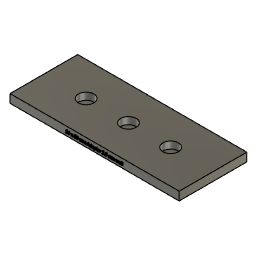
5mm_hydrogel_coverslip_adaptor v2 (Autodesk Fusion 360 design; units mm, degrees)
Autodesk Fusion 360 part; units mm, degrees
sketch "Sketch1" plane through (0, 0, 0) normal (0, 0, 1) x (1, 0, 0)
  line L0 (30, 12) -> (-30, 12)
  line L1 (-30, 12) -> (-30, -12)
  line L2 (-30, -12) -> (30, -12)
  line L3 (30, -12) -> (30, 12)
  line L4 (30, 12) -> (-30, -12) construction
  line L5 (-30, 12) -> (30, -12) construction
  dimension "d1" = 60
  dimension "d2" = 24
  constraint horizontal L0
  constraint perpendicular L0 L1
  constraint parallel L0 L2
  constraint parallel L1 L3
  constraint coincident L4 origin
  constraint coincident L5 origin
  measures "d1" distance of L1.end L2.end
  measures "d2" distance of L0.end L1.end
extrude "Extrude1" add sketch "Sketch1" along normal blind 3
sketch "Sketch2" plane through (0, 0, 3) normal (0, 0, 1) x (-1, 0, 0)
  line L0 (-30, 12) -> (-30, -12)
  line L1 (-30, -12) -> (30, -12)
  line L2 (30, -12) -> (30, 12)
  line L3 (30, 12) -> (-30, 12)
  circle A0 centre (0, 0) radius 2.75
  dimension "d5" = 5.5
  constraint coincident A0.centre origin
  measures "d5" diameter of A0
extrude "Extrude2" cut sketch "Sketch2" against normal blind 2.5 contours A0
sketch "Sketch3" plane through (0, -12, 0) normal (0, -1, 0) x (1, 0, 0)
  line L0 (-30, 0) -> (30, 0)
  line L1 (30, 0) -> (30, 3)
  line L2 (30, 3) -> (-30, 3)
  line L3 (-30, 3) -> (-30, 0)
  line L4 (-9.4664, 1.118) -> (-9.4664, 1)
  line L5 (-9.4664, 1) -> (-10.1274, 1)
  spline S0 degree 2 poles (-10.1274, 1) (-10.1287, 1.0443) (-10.113, 1.0853) knots 0 0 0 1 1 1
  spline S1 degree 2 poles (-10.113, 1.0853) (-10.0878, 1.1528) (-10.0322, 1.2183) knots 0 0 0 1 1 1
  spline S2 degree 2 poles (-10.0322, 1.2183) (-9.9766, 1.2838) (-9.8716, 1.3697) knots 0 0 0 1 1 1
  spline S3 degree 2 poles (-9.8716, 1.3697) (-9.7085, 1.5034) (-9.6512, 1.5815) knots 0 0 0 1 1 1
  spline S4 degree 2 poles (-9.6512, 1.5815) (-9.5939, 1.6596) (-9.5939, 1.7292) knots 0 0 0 1 1 1
  spline S5 degree 2 poles (-9.5939, 1.7292) (-9.5939, 1.8022) (-9.6461, 1.8523) knots 0 0 0 1 1 1
  spline S6 degree 2 poles (-9.6461, 1.8523) (-9.6983, 1.9025) (-9.7822, 1.9025) knots 0 0 0 1 1 1
  spline S7 degree 2 poles (-9.7822, 1.9025) (-9.8709, 1.9025) (-9.9241, 1.8492) knots 0 0 0 1 1 1
  spline S8 degree 2 poles (-9.9241, 1.8492) (-9.9773, 1.796) (-9.978, 1.7019) knots 0 0 0 1 1 1
  line L6 (-9.978, 1.7019) -> (-10.1042, 1.7149)
  spline S9 degree 2 poles (-10.1042, 1.7149) (-10.0912, 1.8561) (-10.0066, 1.9301) knots 0 0 0 1 1 1
  spline S10 degree 2 poles (-10.0066, 1.9301) (-9.922, 2.0041) (-9.7795, 2.0041) knots 0 0 0 1 1 1
  spline S11 degree 2 poles (-9.7795, 2.0041) (-9.6355, 2.0041) (-9.5516, 1.9243) knots 0 0 0 1 1 1
  spline S12 degree 2 poles (-9.5516, 1.9243) (-9.4677, 1.8445) (-9.4677, 1.7265) knots 0 0 0 1 1 1
  spline S13 degree 2 poles (-9.4677, 1.7265) (-9.4677, 1.6664) (-9.4923, 1.6085) knots 0 0 0 1 1 1
  spline S14 degree 2 poles (-9.4923, 1.6085) (-9.5169, 1.5505) (-9.5738, 1.4864) knots 0 0 0 1 1 1
  spline S15 degree 2 poles (-9.5738, 1.4864) (-9.6308, 1.4222) (-9.7631, 1.3104) knots 0 0 0 1 1 1
  spline S16 degree 2 poles (-9.7631, 1.3104) (-9.8736, 1.2176) (-9.905, 1.1845) knots 0 0 0 1 1 1
  spline S17 degree 2 poles (-9.905, 1.1845) (-9.9364, 1.1514) (-9.9568, 1.118) knots 0 0 0 1 1 1
  line L7 (-9.9568, 1.118) -> (-9.4664, 1.118)
  line L8 (-8.9411, 1) -> (-8.9411, 1.2394)
  line L9 (-8.9411, 1.2394) -> (-9.375, 1.2394)
  line L10 (-9.375, 1.2394) -> (-9.375, 1.352)
  line L11 (-9.375, 1.352) -> (-8.9186, 2)
  line L12 (-8.9186, 2) -> (-8.8184, 2)
  line L13 (-8.8184, 2) -> (-8.8184, 1.352)
  line L14 (-8.8184, 1.352) -> (-8.6833, 1.352)
  line L15 (-8.6833, 1.352) -> (-8.6833, 1.2394)
  line L16 (-8.6833, 1.2394) -> (-8.8184, 1.2394)
  line L17 (-8.8184, 1.2394) -> (-8.8184, 1)
  line L18 (-8.8184, 1) -> (-8.9411, 1)
  line L19 (-8.9411, 1.352) -> (-8.9411, 1.8029)
  line L20 (-8.9411, 1.8029) -> (-9.2542, 1.352)
  line L21 (-9.2542, 1.352) -> (-8.9411, 1.352)
  line L22 (-8.2174, 1) -> (-7.9527, 1.3765)
  line L23 (-7.9527, 1.3765) -> (-8.1976, 1.7244)
  line L24 (-8.1976, 1.7244) -> (-8.0441, 1.7244)
  line L25 (-8.0441, 1.7244) -> (-7.933, 1.5546)
  spline S18 degree 2 poles (-7.933, 1.5546) (-7.9016, 1.5061) (-7.8825, 1.4734) knots 0 0 0 1 1 1
  spline S19 degree 2 poles (-7.8825, 1.4734) (-7.8525, 1.5184) (-7.8272, 1.5532) knots 0 0 0 1 1 1
  line L26 (-7.8272, 1.5532) -> (-7.7051, 1.7244)
  line L27 (-7.7051, 1.7244) -> (-7.5585, 1.7244)
  line L28 (-7.5585, 1.7244) -> (-7.8088, 1.3834)
  line L29 (-7.8088, 1.3834) -> (-7.5394, 1)
  line L30 (-7.5394, 1) -> (-7.6901, 1)
  line L31 (-7.6901, 1) -> (-7.8388, 1.2251)
  line L32 (-7.8388, 1.2251) -> (-7.8784, 1.2858)
  line L33 (-7.8784, 1.2858) -> (-8.0687, 1)
  line L34 (-8.0687, 1) -> (-8.2174, 1)
  line L35 (-6.4459, 1.7551) -> (-6.568, 1.7456)
  spline S20 degree 2 poles (-6.568, 1.7456) (-6.5844, 1.8179) (-6.6144, 1.8506) knots 0 0 0 1 1 1
  spline S21 degree 2 poles (-6.6144, 1.8506) (-6.6642, 1.9031) (-6.7372, 1.9031) knots 0 0 0 1 1 1
  spline S22 degree 2 poles (-6.7372, 1.9031) (-6.7958, 1.9031) (-6.8402, 1.8704) knots 0 0 0 1 1 1
  spline S23 degree 2 poles (-6.8402, 1.8704) (-6.8982, 1.8281) (-6.9316, 1.7469) knots 0 0 0 1 1 1
  spline S24 degree 2 poles (-6.9316, 1.7469) (-6.965, 1.6658) (-6.9664, 1.5157) knots 0 0 0 1 1 1
  spline S25 degree 2 poles (-6.9664, 1.5157) (-6.922, 1.5832) (-6.8579, 1.616) knots 0 0 0 1 1 1
  spline S26 degree 2 poles (-6.8579, 1.616) (-6.7938, 1.6487) (-6.7235, 1.6487) knots 0 0 0 1 1 1
  spline S27 degree 2 poles (-6.7235, 1.6487) (-6.6008, 1.6487) (-6.5145, 1.5583) knots 0 0 0 1 1 1
  spline S28 degree 2 poles (-6.5145, 1.5583) (-6.4282, 1.4679) (-6.4282, 1.3247) knots 0 0 0 1 1 1
  spline S29 degree 2 poles (-6.4282, 1.3247) (-6.4282, 1.2306) (-6.4688, 1.1497) knots 0 0 0 1 1 1
  spline S30 degree 2 poles (-6.4688, 1.1497) (-6.5094, 1.0689) (-6.5803, 1.0259) knots 0 0 0 1 1 1
  spline S31 degree 2 poles (-6.5803, 1.0259) (-6.6512, 0.9829) (-6.7413, 0.9829) knots 0 0 0 1 1 1
  spline S32 degree 2 poles (-6.7413, 0.9829) (-6.8948, 0.9829) (-6.9916, 1.0958) knots 0 0 0 1 1 1
  spline S33 degree 2 poles (-6.9916, 1.0958) (-7.0885, 1.2087) (-7.0885, 1.4679) knots 0 0 0 1 1 1
  spline S34 degree 2 poles (-7.0885, 1.4679) (-7.0885, 1.7578) (-6.9814, 1.8895) knots 0 0 0 1 1 1
  spline S35 degree 2 poles (-6.9814, 1.8895) (-6.8879, 2.0041) (-6.7297, 2.0041) knots 0 0 0 1 1 1
  spline S36 degree 2 poles (-6.7297, 2.0041) (-6.6117, 2.0041) (-6.5363, 1.9379) knots 0 0 0 1 1 1
  spline S37 degree 2 poles (-6.5363, 1.9379) (-6.4609, 1.8718) (-6.4459, 1.7551) knots 0 0 0 1 1 1
  spline S38 degree 2 poles (-6.9473, 1.324) (-6.9473, 1.2606) (-6.9203, 1.2026) knots 0 0 0 1 1 1
  spline S39 degree 2 poles (-6.9203, 1.2026) (-6.8934, 1.1446) (-6.845, 1.1143) knots 0 0 0 1 1 1
  spline S40 degree 2 poles (-6.845, 1.1143) (-6.7965, 1.0839) (-6.7433, 1.0839) knots 0 0 0 1 1 1
  spline S41 degree 2 poles (-6.7433, 1.0839) (-6.6656, 1.0839) (-6.6096, 1.1467) knots 0 0 0 1 1 1
  spline S42 degree 2 poles (-6.6096, 1.1467) (-6.5537, 1.2094) (-6.5537, 1.3172) knots 0 0 0 1 1 1
  spline S43 degree 2 poles (-6.5537, 1.3172) (-6.5537, 1.4209) (-6.6089, 1.4806) knots 0 0 0 1 1 1
  spline S44 degree 2 poles (-6.6089, 1.4806) (-6.6642, 1.5402) (-6.7481, 1.5402) knots 0 0 0 1 1 1
  spline S45 degree 2 poles (-6.7481, 1.5402) (-6.8313, 1.5402) (-6.8893, 1.4806) knots 0 0 0 1 1 1
  spline S46 degree 2 poles (-6.8893, 1.4806) (-6.9473, 1.4209) (-6.9473, 1.324) knots 0 0 0 1 1 1
  spline S47 degree 2 poles (-6.3061, 1.4932) (-6.3061, 1.6705) (-6.2696, 1.7786) knots 0 0 0 1 1 1
  spline S48 degree 2 poles (-6.2696, 1.7786) (-6.2331, 1.8868) (-6.1611, 1.9454) knots 0 0 0 1 1 1
  spline S49 degree 2 poles (-6.1611, 1.9454) (-6.0892, 2.0041) (-5.98, 2.0041) knots 0 0 0 1 1 1
  spline S50 degree 2 poles (-5.98, 2.0041) (-5.8995, 2.0041) (-5.8388, 1.9717) knots 0 0 0 1 1 1
  spline S51 degree 2 poles (-5.8388, 1.9717) (-5.7781, 1.9393) (-5.7386, 1.8782) knots 0 0 0 1 1 1
  spline S52 degree 2 poles (-5.7386, 1.8782) (-5.699, 1.8172) (-5.6765, 1.7295) knots 0 0 0 1 1 1
  spline S53 degree 2 poles (-5.6765, 1.7295) (-5.654, 1.6419) (-5.654, 1.4932) knots 0 0 0 1 1 1
  spline S54 degree 2 poles (-5.654, 1.4932) (-5.654, 1.3172) (-5.6901, 1.2091) knots 0 0 0 1 1 1
  spline S55 degree 2 poles (-5.6901, 1.2091) (-5.7263, 1.101) (-5.7982, 1.042) knots 0 0 0 1 1 1
  spline S56 degree 2 poles (-5.7982, 1.042) (-5.8702, 0.9829) (-5.98, 0.9829) knots 0 0 0 1 1 1
  spline S57 degree 2 poles (-5.98, 0.9829) (-6.1246, 0.9829) (-6.2072, 1.0866) knots 0 0 0 1 1 1
  spline S58 degree 2 poles (-6.2072, 1.0866) (-6.3061, 1.2115) (-6.3061, 1.4932) knots 0 0 0 1 1 1
  spline S59 degree 2 poles (-6.1799, 1.4932) (-6.1799, 1.2469) (-6.1222, 1.1654) knots 0 0 0 1 1 1
  spline S60 degree 2 poles (-6.1222, 1.1654) (-6.0646, 1.0839) (-5.98, 1.0839) knots 0 0 0 1 1 1
  spline S61 degree 2 poles (-5.98, 1.0839) (-5.8954, 1.0839) (-5.8378, 1.1658) knots 0 0 0 1 1 1
  spline S62 degree 2 poles (-5.8378, 1.1658) (-5.7802, 1.2476) (-5.7802, 1.4932) knots 0 0 0 1 1 1
  spline S63 degree 2 poles (-5.7802, 1.4932) (-5.7802, 1.7401) (-5.8378, 1.8213) knots 0 0 0 1 1 1
  spline S64 degree 2 poles (-5.8378, 1.8213) (-5.8954, 1.9025) (-5.9814, 1.9025) knots 0 0 0 1 1 1
  spline S65 degree 2 poles (-5.9814, 1.9025) (-6.066, 1.9025) (-6.1165, 1.8308) knots 0 0 0 1 1 1
  spline S66 degree 2 poles (-6.1165, 1.8308) (-6.1799, 1.7394) (-6.1799, 1.4932) knots 0 0 0 1 1 1
  line L36 (-5.1069, 1) -> (-5.1069, 1.7244)
  line L37 (-5.1069, 1.7244) -> (-4.9971, 1.7244)
  line L38 (-4.9971, 1.7244) -> (-4.9971, 1.6228)
  spline S67 degree 2 poles (-4.9971, 1.6228) (-4.963, 1.676) (-4.9064, 1.7084) knots 0 0 0 1 1 1
  spline S68 degree 2 poles (-4.9064, 1.7084) (-4.8497, 1.7408) (-4.7774, 1.7408) knots 0 0 0 1 1 1
  spline S69 degree 2 poles (-4.7774, 1.7408) (-4.6969, 1.7408) (-4.6454, 1.7074) knots 0 0 0 1 1 1
  spline S70 degree 2 poles (-4.6454, 1.7074) (-4.5939, 1.6739) (-4.5728, 1.6139) knots 0 0 0 1 1 1
  spline S71 degree 2 poles (-4.5728, 1.6139) (-4.4868, 1.7408) (-4.3491, 1.7408) knots 0 0 0 1 1 1
  spline S72 degree 2 poles (-4.3491, 1.7408) (-4.2413, 1.7408) (-4.1833, 1.6811) knots 0 0 0 1 1 1
  spline S73 degree 2 poles (-4.1833, 1.6811) (-4.1253, 1.6214) (-4.1253, 1.4973) knots 0 0 0 1 1 1
  line L39 (-4.1253, 1.4973) -> (-4.1253, 1)
  line L40 (-4.1253, 1) -> (-4.2474, 1)
  line L41 (-4.2474, 1) -> (-4.2474, 1.4563)
  spline S74 degree 2 poles (-4.2474, 1.4563) (-4.2474, 1.53) (-4.2594, 1.5624) knots 0 0 0 1 1 1
  spline S75 degree 2 poles (-4.2594, 1.5624) (-4.2713, 1.5948) (-4.3027, 1.6146) knots 0 0 0 1 1 1
  spline S76 degree 2 poles (-4.3027, 1.6146) (-4.334, 1.6344) (-4.3763, 1.6344) knots 0 0 0 1 1 1
  spline S77 degree 2 poles (-4.3763, 1.6344) (-4.4527, 1.6344) (-4.5032, 1.5836) knots 0 0 0 1 1 1
  spline S78 degree 2 poles (-4.5032, 1.5836) (-4.5537, 1.5327) (-4.5537, 1.4209) knots 0 0 0 1 1 1
  line L42 (-4.5537, 1.4209) -> (-4.5537, 1)
  line L43 (-4.5537, 1) -> (-4.6765, 1)
  line L44 (-4.6765, 1) -> (-4.6765, 1.4707)
  spline S79 degree 2 poles (-4.6765, 1.4707) (-4.6765, 1.5525) (-4.7065, 1.5935) knots 0 0 0 1 1 1
  spline S80 degree 2 poles (-4.7065, 1.5935) (-4.7365, 1.6344) (-4.8047, 1.6344) knots 0 0 0 1 1 1
  spline S81 degree 2 poles (-4.8047, 1.6344) (-4.8566, 1.6344) (-4.9006, 1.6071) knots 0 0 0 1 1 1
  spline S82 degree 2 poles (-4.9006, 1.6071) (-4.9446, 1.5798) (-4.9643, 1.5273) knots 0 0 0 1 1 1
  spline S83 degree 2 poles (-4.9643, 1.5273) (-4.9841, 1.4748) (-4.9841, 1.3759) knots 0 0 0 1 1 1
  line L45 (-4.9841, 1.3759) -> (-4.9841, 1)
  line L46 (-4.9841, 1) -> (-5.1069, 1)
  line L47 (-3.9432, 1) -> (-3.9432, 1.7244)
  line L48 (-3.9432, 1.7244) -> (-3.8334, 1.7244)
  line L49 (-3.8334, 1.7244) -> (-3.8334, 1.6228)
  spline S84 degree 2 poles (-3.8334, 1.6228) (-3.7993, 1.676) (-3.7426, 1.7084) knots 0 0 0 1 1 1
  spline S85 degree 2 poles (-3.7426, 1.7084) (-3.686, 1.7408) (-3.6137, 1.7408) knots 0 0 0 1 1 1
  spline S86 degree 2 poles (-3.6137, 1.7408) (-3.5332, 1.7408) (-3.4817, 1.7074) knots 0 0 0 1 1 1
  spline S87 degree 2 poles (-3.4817, 1.7074) (-3.4302, 1.6739) (-3.4091, 1.6139) knots 0 0 0 1 1 1
  spline S88 degree 2 poles (-3.4091, 1.6139) (-3.3231, 1.7408) (-3.1853, 1.7408) knots 0 0 0 1 1 1
  spline S89 degree 2 poles (-3.1853, 1.7408) (-3.0776, 1.7408) (-3.0196, 1.6811) knots 0 0 0 1 1 1
  spline S90 degree 2 poles (-3.0196, 1.6811) (-2.9616, 1.6214) (-2.9616, 1.4973) knots 0 0 0 1 1 1
  line L50 (-2.9616, 1.4973) -> (-2.9616, 1)
  line L51 (-2.9616, 1) -> (-3.0837, 1)
  line L52 (-3.0837, 1) -> (-3.0837, 1.4563)
  spline S91 degree 2 poles (-3.0837, 1.4563) (-3.0837, 1.53) (-3.0956, 1.5624) knots 0 0 0 1 1 1
  spline S92 degree 2 poles (-3.0956, 1.5624) (-3.1076, 1.5948) (-3.139, 1.6146) knots 0 0 0 1 1 1
  spline S93 degree 2 poles (-3.139, 1.6146) (-3.1703, 1.6344) (-3.2126, 1.6344) knots 0 0 0 1 1 1
  spline S94 degree 2 poles (-3.2126, 1.6344) (-3.289, 1.6344) (-3.3395, 1.5836) knots 0 0 0 1 1 1
  spline S95 degree 2 poles (-3.3395, 1.5836) (-3.39, 1.5327) (-3.39, 1.4209) knots 0 0 0 1 1 1
  line L53 (-3.39, 1.4209) -> (-3.39, 1)
  line L54 (-3.39, 1) -> (-3.5128, 1)
  line L55 (-3.5128, 1) -> (-3.5128, 1.4707)
  spline S96 degree 2 poles (-3.5128, 1.4707) (-3.5128, 1.5525) (-3.5428, 1.5935) knots 0 0 0 1 1 1
  spline S97 degree 2 poles (-3.5428, 1.5935) (-3.5728, 1.6344) (-3.641, 1.6344) knots 0 0 0 1 1 1
  spline S98 degree 2 poles (-3.641, 1.6344) (-3.6928, 1.6344) (-3.7368, 1.6071) knots 0 0 0 1 1 1
  spline S99 degree 2 poles (-3.7368, 1.6071) (-3.7808, 1.5798) (-3.8006, 1.5273) knots 0 0 0 1 1 1
  spline S100 degree 2 poles (-3.8006, 1.5273) (-3.8204, 1.4748) (-3.8204, 1.3759) knots 0 0 0 1 1 1
  line L56 (-3.8204, 1.3759) -> (-3.8204, 1)
  line L57 (-3.8204, 1) -> (-3.9432, 1)
  line L58 (-2.5626, 1) -> (-2.1785, 2)
  line L59 (-2.1785, 2) -> (-2.036, 2)
  line L60 (-2.036, 2) -> (-1.6267, 1)
  line L61 (-1.6267, 1) -> (-1.7774, 1)
  line L62 (-1.7774, 1) -> (-1.8941, 1.3029)
  line L63 (-1.8941, 1.3029) -> (-2.3122, 1.3029)
  line L64 (-2.3122, 1.3029) -> (-2.422, 1)
  line L65 (-2.422, 1) -> (-2.5626, 1)
  line L66 (-2.274, 1.4106) -> (-1.935, 1.4106)
  line L67 (-1.935, 1.4106) -> (-2.0394, 1.6876)
  spline S101 degree 2 poles (-2.0394, 1.6876) (-2.0871, 1.8138) (-2.1103, 1.895) knots 0 0 0 1 1 1
  spline S102 degree 2 poles (-2.1103, 1.895) (-2.1294, 1.7988) (-2.1642, 1.704) knots 0 0 0 1 1 1
  line L68 (-2.1642, 1.704) -> (-2.274, 1.4106)
  line L69 (-1.0667, 1) -> (-1.0667, 1.0914)
  spline S103 degree 2 poles (-1.0667, 1.0914) (-1.1355, 0.9836) (-1.2692, 0.9836) knots 0 0 0 1 1 1
  spline S104 degree 2 poles (-1.2692, 0.9836) (-1.3559, 0.9836) (-1.4285, 1.0314) knots 0 0 0 1 1 1
  spline S105 degree 2 poles (-1.4285, 1.0314) (-1.5012, 1.0791) (-1.5411, 1.1647) knots 0 0 0 1 1 1
  spline S106 degree 2 poles (-1.5411, 1.1647) (-1.581, 1.2503) (-1.581, 1.3615) knots 0 0 0 1 1 1
  spline S107 degree 2 poles (-1.581, 1.3615) (-1.581, 1.47) (-1.5448, 1.5583) knots 0 0 0 1 1 1
  spline S108 degree 2 poles (-1.5448, 1.5583) (-1.5087, 1.6467) (-1.4364, 1.6937) knots 0 0 0 1 1 1
  spline S109 degree 2 poles (-1.4364, 1.6937) (-1.3641, 1.7408) (-1.2747, 1.7408) knots 0 0 0 1 1 1
  spline S110 degree 2 poles (-1.2747, 1.7408) (-1.2092, 1.7408) (-1.1581, 1.7132) knots 0 0 0 1 1 1
  spline S111 degree 2 poles (-1.1581, 1.7132) (-1.1069, 1.6855) (-1.0748, 1.6412) knots 0 0 0 1 1 1
  line L70 (-1.0748, 1.6412) -> (-1.0748, 2)
  line L71 (-1.0748, 2) -> (-0.9527, 2)
  line L72 (-0.9527, 2) -> (-0.9527, 1)
  line L73 (-0.9527, 1) -> (-1.0667, 1)
  spline S112 degree 2 poles (-1.4548, 1.3615) (-1.4548, 1.2224) (-1.3961, 1.1535) knots 0 0 0 1 1 1
  spline S113 degree 2 poles (-1.3961, 1.1535) (-1.3375, 1.0846) (-1.2577, 1.0846) knots 0 0 0 1 1 1
  spline S114 degree 2 poles (-1.2577, 1.0846) (-1.1772, 1.0846) (-1.1209, 1.1504) knots 0 0 0 1 1 1
  spline S115 degree 2 poles (-1.1209, 1.1504) (-1.0646, 1.2162) (-1.0646, 1.3513) knots 0 0 0 1 1 1
  spline S116 degree 2 poles (-1.0646, 1.3513) (-1.0646, 1.5) (-1.1219, 1.5696) knots 0 0 0 1 1 1
  spline S117 degree 2 poles (-1.1219, 1.5696) (-1.1792, 1.6392) (-1.2631, 1.6392) knots 0 0 0 1 1 1
  spline S118 degree 2 poles (-1.2631, 1.6392) (-1.345, 1.6392) (-1.3999, 1.5723) knots 0 0 0 1 1 1
  spline S119 degree 2 poles (-1.3999, 1.5723) (-1.4548, 1.5055) (-1.4548, 1.3615) knots 0 0 0 1 1 1
  spline S120 degree 2 poles (-0.287, 1.0894) (-0.3552, 1.0314) (-0.4183, 1.0075) knots 0 0 0 1 1 1
  spline S121 degree 2 poles (-0.4183, 1.0075) (-0.4814, 0.9836) (-0.5537, 0.9836) knots 0 0 0 1 1 1
  spline S122 degree 2 poles (-0.5537, 0.9836) (-0.6731, 0.9836) (-0.7372, 1.042) knots 0 0 0 1 1 1
  spline S123 degree 2 poles (-0.7372, 1.042) (-0.8013, 1.1003) (-0.8013, 1.191) knots 0 0 0 1 1 1
  spline S124 degree 2 poles (-0.8013, 1.191) (-0.8013, 1.2442) (-0.7771, 1.2882) knots 0 0 0 1 1 1
  spline S125 degree 2 poles (-0.7771, 1.2882) (-0.7529, 1.3322) (-0.7137, 1.3588) knots 0 0 0 1 1 1
  spline S126 degree 2 poles (-0.7137, 1.3588) (-0.6744, 1.3854) (-0.6253, 1.399) knots 0 0 0 1 1 1
  spline S127 degree 2 poles (-0.6253, 1.399) (-0.5892, 1.4086) (-0.5162, 1.4175) knots 0 0 0 1 1 1
  spline S128 degree 2 poles (-0.5162, 1.4175) (-0.3675, 1.4352) (-0.2972, 1.4598) knots 0 0 0 1 1 1
  spline S129 degree 2 poles (-0.2972, 1.4598) (-0.2965, 1.485) (-0.2965, 1.4918) knots 0 0 0 1 1 1
  spline S130 degree 2 poles (-0.2965, 1.4918) (-0.2965, 1.5668) (-0.3313, 1.5975) knots 0 0 0 1 1 1
  spline S131 degree 2 poles (-0.3313, 1.5975) (-0.3784, 1.6392) (-0.4712, 1.6392) knots 0 0 0 1 1 1
  spline S132 degree 2 poles (-0.4712, 1.6392) (-0.5578, 1.6392) (-0.5991, 1.6088) knots 0 0 0 1 1 1
  spline S133 degree 2 poles (-0.5991, 1.6088) (-0.6403, 1.5784) (-0.6601, 1.5014) knots 0 0 0 1 1 1
  line L74 (-0.6601, 1.5014) -> (-0.7802, 1.5177)
  spline S134 degree 2 poles (-0.7802, 1.5177) (-0.7638, 1.5948) (-0.7263, 1.6422) knots 0 0 0 1 1 1
  spline S135 degree 2 poles (-0.7263, 1.6422) (-0.6888, 1.6896) (-0.6178, 1.7152) knots 0 0 0 1 1 1
  spline S136 degree 2 poles (-0.6178, 1.7152) (-0.5469, 1.7408) (-0.4534, 1.7408) knots 0 0 0 1 1 1
  spline S137 degree 2 poles (-0.4534, 1.7408) (-0.3607, 1.7408) (-0.3027, 1.719) knots 0 0 0 1 1 1
  spline S138 degree 2 poles (-0.3027, 1.719) (-0.2447, 1.6971) (-0.2174, 1.6641) knots 0 0 0 1 1 1
  spline S139 degree 2 poles (-0.2174, 1.6641) (-0.1901, 1.631) (-0.1792, 1.5805) knots 0 0 0 1 1 1
  spline S140 degree 2 poles (-0.1792, 1.5805) (-0.1731, 1.5491) (-0.1731, 1.4673) knots 0 0 0 1 1 1
  line L75 (-0.1731, 1.4673) -> (-0.1731, 1.3035)
  spline S141 degree 2 poles (-0.1731, 1.3035) (-0.1731, 1.1323) (-0.1652, 1.087) knots 0 0 0 1 1 1
  spline S142 degree 2 poles (-0.1652, 1.087) (-0.1574, 1.0416) (-0.1342, 1) knots 0 0 0 1 1 1
  line L76 (-0.1342, 1) -> (-0.2624, 1)
  spline S143 degree 2 poles (-0.2624, 1) (-0.2815, 1.0382) (-0.287, 1.0894) knots 0 0 0 1 1 1
  spline S144 degree 2 poles (-0.2972, 1.3636) (-0.3641, 1.3363) (-0.4978, 1.3172) knots 0 0 0 1 1 1
  spline S145 degree 2 poles (-0.4978, 1.3172) (-0.5735, 1.3063) (-0.6049, 1.2926) knots 0 0 0 1 1 1
  spline S146 degree 2 poles (-0.6049, 1.2926) (-0.6362, 1.279) (-0.6533, 1.2527) knots 0 0 0 1 1 1
  spline S147 degree 2 poles (-0.6533, 1.2527) (-0.6703, 1.2265) (-0.6703, 1.1944) knots 0 0 0 1 1 1
  spline S148 degree 2 poles (-0.6703, 1.1944) (-0.6703, 1.1453) (-0.6332, 1.1126) knots 0 0 0 1 1 1
  spline S149 degree 2 poles (-0.6332, 1.1126) (-0.596, 1.0798) (-0.5244, 1.0798) knots 0 0 0 1 1 1
  spline S150 degree 2 poles (-0.5244, 1.0798) (-0.4534, 1.0798) (-0.3982, 1.1108) knots 0 0 0 1 1 1
  spline S151 degree 2 poles (-0.3982, 1.1108) (-0.3429, 1.1419) (-0.317, 1.1958) knots 0 0 0 1 1 1
  spline S152 degree 2 poles (-0.317, 1.1958) (-0.2972, 1.2374) (-0.2972, 1.3186) knots 0 0 0 1 1 1
  line L77 (-0.2972, 1.3186) -> (-0.2972, 1.3636)
  line L78 (0.0172, 0.7224) -> (0.0172, 1.7244)
  line L79 (0.0172, 1.7244) -> (0.1291, 1.7244)
  line L80 (0.1291, 1.7244) -> (0.1291, 1.6303)
  spline S153 degree 2 poles (0.1291, 1.6303) (0.1687, 1.6855) (0.2185, 1.7132) knots 0 0 0 1 1 1
  spline S154 degree 2 poles (0.2185, 1.7132) (0.2683, 1.7408) (0.3392, 1.7408) knots 0 0 0 1 1 1
  spline S155 degree 2 poles (0.3392, 1.7408) (0.432, 1.7408) (0.5029, 1.693) knots 0 0 0 1 1 1
  spline S156 degree 2 poles (0.5029, 1.693) (0.5739, 1.6453) (0.61, 1.5583) knots 0 0 0 1 1 1
  spline S157 degree 2 poles (0.61, 1.5583) (0.6462, 1.4714) (0.6462, 1.3677) knots 0 0 0 1 1 1
  spline S158 degree 2 poles (0.6462, 1.3677) (0.6462, 1.2565) (0.6063, 1.1675) knots 0 0 0 1 1 1
  spline S159 degree 2 poles (0.6063, 1.1675) (0.5664, 1.0784) (0.4903, 1.031) knots 0 0 0 1 1 1
  spline S160 degree 2 poles (0.4903, 1.031) (0.4142, 0.9836) (0.3303, 0.9836) knots 0 0 0 1 1 1
  spline S161 degree 2 poles (0.3303, 0.9836) (0.269, 0.9836) (0.2202, 1.0095) knots 0 0 0 1 1 1
  spline S162 degree 2 poles (0.2202, 1.0095) (0.1714, 1.0355) (0.14, 1.075) knots 0 0 0 1 1 1
  line L81 (0.14, 1.075) -> (0.14, 0.7224)
  line L82 (0.14, 0.7224) -> (0.0172, 0.7224)
  spline S163 degree 2 poles (0.1284, 1.3581) (0.1284, 1.2183) (0.1851, 1.1514) knots 0 0 0 1 1 1
  spline S164 degree 2 poles (0.1851, 1.1514) (0.2417, 1.0846) (0.3222, 1.0846) knots 0 0 0 1 1 1
  spline S165 degree 2 poles (0.3222, 1.0846) (0.404, 1.0846) (0.4623, 1.1538) knots 0 0 0 1 1 1
  spline S166 degree 2 poles (0.4623, 1.1538) (0.5207, 1.2231) (0.5207, 1.3683) knots 0 0 0 1 1 1
  spline S167 degree 2 poles (0.5207, 1.3683) (0.5207, 1.5068) (0.4637, 1.5757) knots 0 0 0 1 1 1
  spline S168 degree 2 poles (0.4637, 1.5757) (0.4067, 1.6446) (0.3276, 1.6446) knots 0 0 0 1 1 1
  spline S169 degree 2 poles (0.3276, 1.6446) (0.2492, 1.6446) (0.1888, 1.5713) knots 0 0 0 1 1 1
  spline S170 degree 2 poles (0.1888, 1.5713) (0.1284, 1.498) (0.1284, 1.3581) knots 0 0 0 1 1 1
  line L83 (1.0623, 1.1098) -> (1.08, 1.0014)
  spline S171 degree 2 poles (1.08, 1.0014) (1.0282, 0.9905) (0.9872, 0.9905) knots 0 0 0 1 1 1
  spline S172 degree 2 poles (0.9872, 0.9905) (0.9204, 0.9905) (0.8836, 1.0116) knots 0 0 0 1 1 1
  spline S173 degree 2 poles (0.8836, 1.0116) (0.8467, 1.0327) (0.8317, 1.0672) knots 0 0 0 1 1 1
  spline S174 degree 2 poles (0.8317, 1.0672) (0.8167, 1.1016) (0.8167, 1.2121) knots 0 0 0 1 1 1
  line L84 (0.8167, 1.2121) -> (0.8167, 1.6289)
  line L85 (0.8167, 1.6289) -> (0.7267, 1.6289)
  line L86 (0.7267, 1.6289) -> (0.7267, 1.7244)
  line L87 (0.7267, 1.7244) -> (0.8167, 1.7244)
  line L88 (0.8167, 1.7244) -> (0.8167, 1.9038)
  line L89 (0.8167, 1.9038) -> (0.9388, 1.9775)
  line L90 (0.9388, 1.9775) -> (0.9388, 1.7244)
  line L91 (0.9388, 1.7244) -> (1.0623, 1.7244)
  line L92 (1.0623, 1.7244) -> (1.0623, 1.6289)
  line L93 (1.0623, 1.6289) -> (0.9388, 1.6289)
  line L94 (0.9388, 1.6289) -> (0.9388, 1.2053)
  spline S175 degree 2 poles (0.9388, 1.2053) (0.9388, 1.1528) (0.9453, 1.1378) knots 0 0 0 1 1 1
  spline S176 degree 2 poles (0.9453, 1.1378) (0.9518, 1.1228) (0.9664, 1.1139) knots 0 0 0 1 1 1
  spline S177 degree 2 poles (0.9664, 1.1139) (0.9811, 1.105) (1.0084, 1.105) knots 0 0 0 1 1 1
  spline S178 degree 2 poles (1.0084, 1.105) (1.0288, 1.105) (1.0623, 1.1098) knots 0 0 0 1 1 1
  spline S179 degree 2 poles (1.1366, 1.3622) (1.1366, 1.5634) (1.2485, 1.6603) knots 0 0 0 1 1 1
  spline S180 degree 2 poles (1.2485, 1.6603) (1.3419, 1.7408) (1.4763, 1.7408) knots 0 0 0 1 1 1
  spline S181 degree 2 poles (1.4763, 1.7408) (1.6257, 1.7408) (1.7205, 1.6429) knots 0 0 0 1 1 1
  spline S182 degree 2 poles (1.7205, 1.6429) (1.8153, 1.545) (1.8153, 1.3724) knots 0 0 0 1 1 1
  spline S183 degree 2 poles (1.8153, 1.3724) (1.8153, 1.2326) (1.7734, 1.1525) knots 0 0 0 1 1 1
  spline S184 degree 2 poles (1.7734, 1.1525) (1.7314, 1.0723) (1.6513, 1.028) knots 0 0 0 1 1 1
  spline S185 degree 2 poles (1.6513, 1.028) (1.5711, 0.9836) (1.4763, 0.9836) knots 0 0 0 1 1 1
  spline S186 degree 2 poles (1.4763, 0.9836) (1.3242, 0.9836) (1.2304, 1.0812) knots 0 0 0 1 1 1
  spline S187 degree 2 poles (1.2304, 1.0812) (1.1366, 1.1787) (1.1366, 1.3622) knots 0 0 0 1 1 1
  spline S188 degree 2 poles (1.2628, 1.3622) (1.2628, 1.2231) (1.3235, 1.1538) knots 0 0 0 1 1 1
  spline S189 degree 2 poles (1.3235, 1.1538) (1.3842, 1.0846) (1.4763, 1.0846) knots 0 0 0 1 1 1
  spline S190 degree 2 poles (1.4763, 1.0846) (1.5677, 1.0846) (1.6284, 1.1542) knots 0 0 0 1 1 1
  spline S191 degree 2 poles (1.6284, 1.1542) (1.6891, 1.2237) (1.6891, 1.3663) knots 0 0 0 1 1 1
  spline S192 degree 2 poles (1.6891, 1.3663) (1.6891, 1.5007) (1.6281, 1.5699) knots 0 0 0 1 1 1
  spline S193 degree 2 poles (1.6281, 1.5699) (1.567, 1.6392) (1.4763, 1.6392) knots 0 0 0 1 1 1
  spline S194 degree 2 poles (1.4763, 1.6392) (1.3842, 1.6392) (1.3235, 1.5703) knots 0 0 0 1 1 1
  spline S195 degree 2 poles (1.3235, 1.5703) (1.2628, 1.5014) (1.2628, 1.3622) knots 0 0 0 1 1 1
  line L95 (1.9579, 1) -> (1.9579, 1.7244)
  line L96 (1.9579, 1.7244) -> (2.0684, 1.7244)
  line L97 (2.0684, 1.7244) -> (2.0684, 1.6146)
  spline S196 degree 2 poles (2.0684, 1.6146) (2.1107, 1.6917) (2.1465, 1.7162) knots 0 0 0 1 1 1
  spline S197 degree 2 poles (2.1465, 1.7162) (2.1823, 1.7408) (2.2253, 1.7408) knots 0 0 0 1 1 1
  spline S198 degree 2 poles (2.2253, 1.7408) (2.2874, 1.7408) (2.3515, 1.7012) knots 0 0 0 1 1 1
  line L98 (2.3515, 1.7012) -> (2.3092, 1.5873)
  spline S199 degree 2 poles (2.3092, 1.5873) (2.2642, 1.6139) (2.2192, 1.6139) knots 0 0 0 1 1 1
  spline S200 degree 2 poles (2.2192, 1.6139) (2.1789, 1.6139) (2.1469, 1.5897) knots 0 0 0 1 1 1
  spline S201 degree 2 poles (2.1469, 1.5897) (2.1148, 1.5655) (2.1011, 1.5225) knots 0 0 0 1 1 1
  spline S202 degree 2 poles (2.1011, 1.5225) (2.0807, 1.457) (2.0807, 1.3793) knots 0 0 0 1 1 1
  line L99 (2.0807, 1.3793) -> (2.0807, 1)
  line L100 (2.0807, 1) -> (1.9579, 1)
  line L101 (3.4238, 1.118) -> (3.4238, 1)
  line L102 (3.4238, 1) -> (2.7628, 1)
  spline S203 degree 2 poles (2.7628, 1) (2.7614, 1.0443) (2.7771, 1.0853) knots 0 0 0 1 1 1
  spline S204 degree 2 poles (2.7771, 1.0853) (2.8024, 1.1528) (2.858, 1.2183) knots 0 0 0 1 1 1
  spline S205 degree 2 poles (2.858, 1.2183) (2.9136, 1.2838) (3.0186, 1.3697) knots 0 0 0 1 1 1
  spline S206 degree 2 poles (3.0186, 1.3697) (3.1816, 1.5034) (3.2389, 1.5815) knots 0 0 0 1 1 1
  spline S207 degree 2 poles (3.2389, 1.5815) (3.2962, 1.6596) (3.2962, 1.7292) knots 0 0 0 1 1 1
  spline S208 degree 2 poles (3.2962, 1.7292) (3.2962, 1.8022) (3.2441, 1.8523) knots 0 0 0 1 1 1
  spline S209 degree 2 poles (3.2441, 1.8523) (3.1919, 1.9025) (3.108, 1.9025) knots 0 0 0 1 1 1
  spline S210 degree 2 poles (3.108, 1.9025) (3.0193, 1.9025) (2.9661, 1.8492) knots 0 0 0 1 1 1
  spline S211 degree 2 poles (2.9661, 1.8492) (2.9129, 1.796) (2.9122, 1.7019) knots 0 0 0 1 1 1
  line L103 (2.9122, 1.7019) -> (2.786, 1.7149)
  spline S212 degree 2 poles (2.786, 1.7149) (2.799, 1.8561) (2.8836, 1.9301) knots 0 0 0 1 1 1
  spline S213 degree 2 poles (2.8836, 1.9301) (2.9681, 2.0041) (3.1107, 2.0041) knots 0 0 0 1 1 1
  spline S214 degree 2 poles (3.1107, 2.0041) (3.2546, 2.0041) (3.3385, 1.9243) knots 0 0 0 1 1 1
  spline S215 degree 2 poles (3.3385, 1.9243) (3.4224, 1.8445) (3.4224, 1.7265) knots 0 0 0 1 1 1
  spline S216 degree 2 poles (3.4224, 1.7265) (3.4224, 1.6664) (3.3979, 1.6085) knots 0 0 0 1 1 1
  spline S217 degree 2 poles (3.3979, 1.6085) (3.3733, 1.5505) (3.3164, 1.4864) knots 0 0 0 1 1 1
  spline S218 degree 2 poles (3.3164, 1.4864) (3.2594, 1.4222) (3.1271, 1.3104) knots 0 0 0 1 1 1
  spline S219 degree 2 poles (3.1271, 1.3104) (3.0166, 1.2176) (2.9852, 1.1845) knots 0 0 0 1 1 1
  spline S220 degree 2 poles (2.9852, 1.1845) (2.9538, 1.1514) (2.9333, 1.118) knots 0 0 0 1 1 1
  line L104 (2.9333, 1.118) -> (3.4238, 1.118)
  line L105 (3.6243, 1) -> (3.6243, 1.1398)
  line L106 (3.6243, 1.1398) -> (3.7642, 1.1398)
  line L107 (3.7642, 1.1398) -> (3.7642, 1)
  line L108 (3.7642, 1) -> (3.6243, 1)
  line L109 (3.9436, 1.2619) -> (4.0725, 1.2729)
  spline S221 degree 2 poles (4.0725, 1.2729) (4.0868, 1.1787) (4.139, 1.1313) knots 0 0 0 1 1 1
  spline S222 degree 2 poles (4.139, 1.1313) (4.1912, 1.0839) (4.2649, 1.0839) knots 0 0 0 1 1 1
  spline S223 degree 2 poles (4.2649, 1.0839) (4.3535, 1.0839) (4.4149, 1.1508) knots 0 0 0 1 1 1
  spline S224 degree 2 poles (4.4149, 1.1508) (4.4763, 1.2176) (4.4763, 1.3281) knots 0 0 0 1 1 1
  spline S225 degree 2 poles (4.4763, 1.3281) (4.4763, 1.4332) (4.4173, 1.4939) knots 0 0 0 1 1 1
  spline S226 degree 2 poles (4.4173, 1.4939) (4.3583, 1.5546) (4.2628, 1.5546) knots 0 0 0 1 1 1
  spline S227 degree 2 poles (4.2628, 1.5546) (4.2035, 1.5546) (4.1557, 1.5276) knots 0 0 0 1 1 1
  spline S228 degree 2 poles (4.1557, 1.5276) (4.108, 1.5007) (4.0807, 1.4577) knots 0 0 0 1 1 1
  line L110 (4.0807, 1.4577) -> (3.9654, 1.4727)
  line L111 (3.9654, 1.4727) -> (4.0623, 1.9864)
  line L112 (4.0623, 1.9864) -> (4.5595, 1.9864)
  line L113 (4.5595, 1.9864) -> (4.5595, 1.869)
  line L114 (4.5595, 1.869) -> (4.1605, 1.869)
  line L115 (4.1605, 1.869) -> (4.1066, 1.6003)
  spline S229 degree 2 poles (4.1066, 1.6003) (4.1966, 1.663) (4.2956, 1.663) knots 0 0 0 1 1 1
  spline S230 degree 2 poles (4.2956, 1.663) (4.4265, 1.663) (4.5166, 1.5723) knots 0 0 0 1 1 1
  spline S231 degree 2 poles (4.5166, 1.5723) (4.6066, 1.4816) (4.6066, 1.339) knots 0 0 0 1 1 1
  spline S232 degree 2 poles (4.6066, 1.339) (4.6066, 1.2033) (4.5275, 1.1044) knots 0 0 0 1 1 1
  spline S233 degree 2 poles (4.5275, 1.1044) (4.4313, 0.9829) (4.2649, 0.9829) knots 0 0 0 1 1 1
  spline S234 degree 2 poles (4.2649, 0.9829) (4.1284, 0.9829) (4.0421, 1.0593) knots 0 0 0 1 1 1
  spline S235 degree 2 poles (4.0421, 1.0593) (3.9559, 1.1357) (3.9436, 1.2619) knots 0 0 0 1 1 1
  line L116 (5.1428, 1) -> (5.1428, 1.7244)
  line L117 (5.1428, 1.7244) -> (5.2526, 1.7244)
  line L118 (5.2526, 1.7244) -> (5.2526, 1.6228)
  spline S236 degree 2 poles (5.2526, 1.6228) (5.2867, 1.676) (5.3433, 1.7084) knots 0 0 0 1 1 1
  spline S237 degree 2 poles (5.3433, 1.7084) (5.3999, 1.7408) (5.4722, 1.7408) knots 0 0 0 1 1 1
  spline S238 degree 2 poles (5.4722, 1.7408) (5.5527, 1.7408) (5.6042, 1.7074) knots 0 0 0 1 1 1
  spline S239 degree 2 poles (5.6042, 1.7074) (5.6557, 1.6739) (5.6769, 1.6139) knots 0 0 0 1 1 1
  spline S240 degree 2 poles (5.6769, 1.6139) (5.7628, 1.7408) (5.9006, 1.7408) knots 0 0 0 1 1 1
  spline S241 degree 2 poles (5.9006, 1.7408) (6.0084, 1.7408) (6.0664, 1.6811) knots 0 0 0 1 1 1
  spline S242 degree 2 poles (6.0664, 1.6811) (6.1243, 1.6214) (6.1243, 1.4973) knots 0 0 0 1 1 1
  line L119 (6.1243, 1.4973) -> (6.1243, 1)
  line L120 (6.1243, 1) -> (6.0022, 1)
  line L121 (6.0022, 1) -> (6.0022, 1.4563)
  spline S243 degree 2 poles (6.0022, 1.4563) (6.0022, 1.53) (5.9903, 1.5624) knots 0 0 0 1 1 1
  spline S244 degree 2 poles (5.9903, 1.5624) (5.9784, 1.5948) (5.947, 1.6146) knots 0 0 0 1 1 1
  spline S245 degree 2 poles (5.947, 1.6146) (5.9156, 1.6344) (5.8733, 1.6344) knots 0 0 0 1 1 1
  spline S246 degree 2 poles (5.8733, 1.6344) (5.7969, 1.6344) (5.7464, 1.5836) knots 0 0 0 1 1 1
  spline S247 degree 2 poles (5.7464, 1.5836) (5.696, 1.5327) (5.696, 1.4209) knots 0 0 0 1 1 1
  line L122 (5.696, 1.4209) -> (5.696, 1)
  line L123 (5.696, 1) -> (5.5732, 1)
  line L124 (5.5732, 1) -> (5.5732, 1.4707)
  spline S248 degree 2 poles (5.5732, 1.4707) (5.5732, 1.5525) (5.5432, 1.5935) knots 0 0 0 1 1 1
  spline S249 degree 2 poles (5.5432, 1.5935) (5.5132, 1.6344) (5.4449, 1.6344) knots 0 0 0 1 1 1
  spline S250 degree 2 poles (5.4449, 1.6344) (5.3931, 1.6344) (5.3491, 1.6071) knots 0 0 0 1 1 1
  spline S251 degree 2 poles (5.3491, 1.6071) (5.3051, 1.5798) (5.2853, 1.5273) knots 0 0 0 1 1 1
  spline S252 degree 2 poles (5.2853, 1.5273) (5.2655, 1.4748) (5.2655, 1.3759) knots 0 0 0 1 1 1
  line L125 (5.2655, 1.3759) -> (5.2655, 1)
  line L126 (5.2655, 1) -> (5.1428, 1)
  line L127 (6.3065, 1) -> (6.3065, 1.7244)
  line L128 (6.3065, 1.7244) -> (6.4163, 1.7244)
  line L129 (6.4163, 1.7244) -> (6.4163, 1.6228)
  spline S253 degree 2 poles (6.4163, 1.6228) (6.4504, 1.676) (6.507, 1.7084) knots 0 0 0 1 1 1
  spline S254 degree 2 poles (6.507, 1.7084) (6.5636, 1.7408) (6.6359, 1.7408) knots 0 0 0 1 1 1
  spline S255 degree 2 poles (6.6359, 1.7408) (6.7164, 1.7408) (6.7679, 1.7074) knots 0 0 0 1 1 1
  spline S256 degree 2 poles (6.7679, 1.7074) (6.8194, 1.6739) (6.8406, 1.6139) knots 0 0 0 1 1 1
  spline S257 degree 2 poles (6.8406, 1.6139) (6.9265, 1.7408) (7.0643, 1.7408) knots 0 0 0 1 1 1
  spline S258 degree 2 poles (7.0643, 1.7408) (7.1721, 1.7408) (7.2301, 1.6811) knots 0 0 0 1 1 1
  spline S259 degree 2 poles (7.2301, 1.6811) (7.2881, 1.6214) (7.2881, 1.4973) knots 0 0 0 1 1 1
  line L130 (7.2881, 1.4973) -> (7.2881, 1)
  line L131 (7.2881, 1) -> (7.1659, 1)
  line L132 (7.1659, 1) -> (7.1659, 1.4563)
  spline S260 degree 2 poles (7.1659, 1.4563) (7.1659, 1.53) (7.154, 1.5624) knots 0 0 0 1 1 1
  spline S261 degree 2 poles (7.154, 1.5624) (7.1421, 1.5948) (7.1107, 1.6146) knots 0 0 0 1 1 1
  spline S262 degree 2 poles (7.1107, 1.6146) (7.0793, 1.6344) (7.037, 1.6344) knots 0 0 0 1 1 1
  spline S263 degree 2 poles (7.037, 1.6344) (6.9606, 1.6344) (6.9102, 1.5836) knots 0 0 0 1 1 1
  spline S264 degree 2 poles (6.9102, 1.5836) (6.8597, 1.5327) (6.8597, 1.4209) knots 0 0 0 1 1 1
  line L133 (6.8597, 1.4209) -> (6.8597, 1)
  line L134 (6.8597, 1) -> (6.7369, 1)
  line L135 (6.7369, 1) -> (6.7369, 1.4707)
  spline S265 degree 2 poles (6.7369, 1.4707) (6.7369, 1.5525) (6.7069, 1.5935) knots 0 0 0 1 1 1
  spline S266 degree 2 poles (6.7069, 1.5935) (6.6769, 1.6344) (6.6087, 1.6344) knots 0 0 0 1 1 1
  spline S267 degree 2 poles (6.6087, 1.6344) (6.5568, 1.6344) (6.5128, 1.6071) knots 0 0 0 1 1 1
  spline S268 degree 2 poles (6.5128, 1.6071) (6.4688, 1.5798) (6.449, 1.5273) knots 0 0 0 1 1 1
  spline S269 degree 2 poles (6.449, 1.5273) (6.4293, 1.4748) (6.4293, 1.3759) knots 0 0 0 1 1 1
  line L136 (6.4293, 1.3759) -> (6.4293, 1)
  line L137 (6.4293, 1) -> (6.3065, 1)
  line L138 (7.992, 1) -> (7.7703, 1.7244)
  line L139 (7.7703, 1.7244) -> (7.8972, 1.7244)
  line L140 (7.8972, 1.7244) -> (8.0125, 1.3063)
  line L141 (8.0125, 1.3063) -> (8.0554, 1.1508)
  spline S270 degree 2 poles (8.0554, 1.1508) (8.0582, 1.1623) (8.093, 1.3001) knots 0 0 0 1 1 1
  line L142 (8.093, 1.3001) -> (8.2082, 1.7244)
  line L143 (8.2082, 1.7244) -> (8.3344, 1.7244)
  line L144 (8.3344, 1.7244) -> (8.4429, 1.3042)
  line L145 (8.4429, 1.3042) -> (8.479, 1.1658)
  line L146 (8.479, 1.1658) -> (8.5207, 1.3056)
  line L147 (8.5207, 1.3056) -> (8.6448, 1.7244)
  line L148 (8.6448, 1.7244) -> (8.7642, 1.7244)
  line L149 (8.7642, 1.7244) -> (8.5377, 1)
  line L150 (8.5377, 1) -> (8.4102, 1)
  line L151 (8.4102, 1) -> (8.2949, 1.4338)
  line L152 (8.2949, 1.4338) -> (8.2669, 1.5573)
  line L153 (8.2669, 1.5573) -> (8.1202, 1)
  line L154 (8.1202, 1) -> (7.992, 1)
  line L155 (9.3631, 1.2333) -> (9.49, 1.2176)
  spline S271 degree 2 poles (9.49, 1.2176) (9.46, 1.1064) (9.3788, 1.045) knots 0 0 0 1 1 1
  spline S272 degree 2 poles (9.3788, 1.045) (9.2976, 0.9836) (9.1714, 0.9836) knots 0 0 0 1 1 1
  spline S273 degree 2 poles (9.1714, 0.9836) (9.0125, 0.9836) (8.9194, 1.0815) knots 0 0 0 1 1 1
  spline S274 degree 2 poles (8.9194, 1.0815) (8.8263, 1.1794) (8.8263, 1.3561) knots 0 0 0 1 1 1
  spline S275 degree 2 poles (8.8263, 1.3561) (8.8263, 1.5389) (8.9204, 1.6398) knots 0 0 0 1 1 1
  spline S276 degree 2 poles (8.9204, 1.6398) (9.0145, 1.7408) (9.1646, 1.7408) knots 0 0 0 1 1 1
  spline S277 degree 2 poles (9.1646, 1.7408) (9.3099, 1.7408) (9.402, 1.6419) knots 0 0 0 1 1 1
  spline S278 degree 2 poles (9.402, 1.6419) (9.4941, 1.543) (9.4941, 1.3636) knots 0 0 0 1 1 1
  spline S279 degree 2 poles (9.4941, 1.3636) (9.4941, 1.3527) (9.4934, 1.3308) knots 0 0 0 1 1 1
  line L156 (9.4934, 1.3308) -> (8.9531, 1.3308)
  spline S280 degree 2 poles (8.9531, 1.3308) (8.9599, 1.2115) (9.0207, 1.148) knots 0 0 0 1 1 1
  spline S281 degree 2 poles (9.0207, 1.148) (9.0814, 1.0846) (9.1721, 1.0846) knots 0 0 0 1 1 1
  spline S282 degree 2 poles (9.1721, 1.0846) (9.2396, 1.0846) (9.2874, 1.1201) knots 0 0 0 1 1 1
  spline S283 degree 2 poles (9.2874, 1.1201) (9.3351, 1.1555) (9.3631, 1.2333) knots 0 0 0 1 1 1
  line L157 (8.9599, 1.4318) -> (9.3644, 1.4318)
  spline S284 degree 2 poles (9.3644, 1.4318) (9.3563, 1.5232) (9.3181, 1.5689) knots 0 0 0 1 1 1
  spline S285 degree 2 poles (9.3181, 1.5689) (9.2594, 1.6398) (9.166, 1.6398) knots 0 0 0 1 1 1
  spline S286 degree 2 poles (9.166, 1.6398) (9.0814, 1.6398) (9.0237, 1.5832) knots 0 0 0 1 1 1
  spline S287 degree 2 poles (9.0237, 1.5832) (8.9661, 1.5266) (8.9599, 1.4318) knots 0 0 0 1 1 1
  line L158 (9.6414, 1) -> (9.6414, 2)
  line L159 (9.6414, 2) -> (9.7642, 2)
  line L160 (9.7642, 2) -> (9.7642, 1)
  line L161 (9.7642, 1) -> (9.6414, 1)
  line L162 (9.9518, 1) -> (9.9518, 2)
  line L163 (9.9518, 2) -> (10.0745, 2)
  line L164 (10.0745, 2) -> (10.0745, 1)
  line L165 (10.0745, 1) -> (9.9518, 1)
extrude "Extrude3" add sketch "Sketch3" along normal blind 0.3 contours L4 L5 S0 S1 S2 S3 S4 S5 S6 S7 S8 L6 S9 S10 S11 S12 S13 S14 S15 S16 S17 L7 | L8 L9 L10 L11 L12 L13 L14 L15 L16 L17 L18 | L22 L23 L24 L25 S18 S19 L26 L27 L28 L29 L30 L31 L32 L33 L34 | L35 S20 S21 S22 S23 S24 S25 S26 S27 S28 S29 S30 S31 S32 S33 S34 S35 S36 S37 | S47 S48 S49 S50 S51 S52 S53 S54 S55 S56 S57 S58 | L36 L37 L38 S67 S68 S69 S70 S71 S72 S73 L39 L40 L41 S74 S75 S76 S77 S78 L42 L43 L44 S79 S80 S81 S82 S83 L45 L46 | L47 L48 L49 S84 S85 S86 S87 S88 S89 S90 L50 L51 L52 S91 S92 S93 S94 S95 L53 L54 L55 S96 S97 S98 S99 S100 L56 L57 | L58 L59 L60 L61 L62 L63 L64 L65 | L69 S103 S104 S105 S106 S107 S108 S109 S110 S111 L70 L71 L72 L73 | S120 S121 S122 S123 S124 S125 S126 S127 S128 S129 S130 S131 S132 S133 L74 S134 S135 S136 S137 S138 S139 S140 L75 S141 S142 L76 S143 | L78 L79 L80 S153 S154 S155 S156 S157 S158 S159 S160 S161 S162 L81 L82 | L83 S171 S172 S173 S174 L84 L85 L86 L87 L88 L89 L90 L91 L92 L93 L94 S175 S176 S177 S178 | S179 S180 S181 S182 S183 S184 S185 S186 S187 | L95 L96 L97 S196 S197 S198 L98 S199 S200 S201 S202 L99 L100 | L101 L102 S203 S204 S205 S206 S207 S208 S209 S210 S211 L103 S212 S213 S214 S215 S216 S217 S218 S219 S220 L104 | L105 L106 L107 L108 | L109 S221 S222 S223 S224 S225 S226 S227 S228 L110 L111 L112 L113 L114 L115 S229 S230 S231 S232 S233 S234 S235 | L116 L117 L118 S236 S237 S238 S239 S240 S241 S242 L119 L120 L121 S243 S244 S245 S246 S247 L122 L123 L124 S248 S249 S250 S251 S252 L125 L126 | L127 L128 L129 S253 S254 S255 S256 S257 S258 S259 L130 L131 L132 S260 S261 S262 S263 S264 L133 L134 L135 S265 S266 S267 S268 S269 L136 L137 | L138 L139 L140 L141 S270 L142 L143 L144 L145 L146 L147 L148 L149 L150 L151 L152 L153 L154 | L155 S271 S272 S273 S274 S275 S276 S277 S278 S279 L156 S280 S281 S282 S283 | L158 L159 L160 L161 | L162 L163 L164 L165
pattern_linear "R-Pattern1" count 3 spacing 15 along (-1, 0, 0) both ways of "Extrude2"
